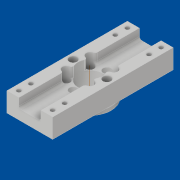
# Autodesk Inventor part: 401-flange
Saved by Autodesk Inventor 2018 (Build 220112000, 112)
## iProperties
Created: 2020-06-11
Part Number: 401-flange
Material: Generic
Document SubType Name: Modeling
Designer: Bunny320
Density: 1 g/cm^3
Appearance: Default
Author: Bunny320
Autodesk Inventor part; units mm, degrees
ref_plane "YZ Plane" through (0, 0, 0) normal (1, 0, 0) x (0, 1, 0)
ref_plane "XZ Plane" through (0, 0, 0) normal (0, 1, 0) x (-1, 0, 0)
ref_plane "XY Plane" through (0, 0, 0) normal (0, 0, 1) x (1, 0, 0)
sketch "Sketch1" plane through (0, 0, 0) normal (0, 0, 1) x (1, 0, 0)
  circle A0 centre (0, 0) radius 17.5
  dimension "d0" = 35
  constraints: 1 centre point, 1 coincident
  measures "d0" diameter of A0
extrude "Extrusion1" add sketch "Sketch1" along normal blind 5
sketch "Sketch2" plane through (0, 0, 5) normal (0, 0, 1) x (1, 0, 0)
  line L0 (-19, -50) -> (19, -50)
  line L1 (19, -50) -> (19, 50)
  line L2 (19, 50) -> (-19, 50)
  line L3 (-19, 50) -> (-19, -50)
  line L4 (-19, -50) -> (19, 50) construction
  line L5 (19, -50) -> (-19, 50) construction
  point P0 (0, 0)
  dimension "d3" = 38
  dimension "d4" = 100
  constraints: 12 end point, 2 midpoint, 2 parallel, 1 horizontal, 1 perpendicular
  measures "d3" distance of L1.end L2.end
  measures "d4" distance of L0.end L1.end
extrude "Extrusion2" add sketch "Sketch2" along normal blind 16
sketch "Sketch3" plane through (0, 0, 21) normal (0, 0, 1) x (1, 0, 0)
  point P0 (0, 0)
  point P1 (14, 0)
  dimension "d7" = 14
  constraints: 1 horizontal alignment
  measures "d7" distance of point (0, 0) point (14, 0)
hole "Hole1" at (14, 0, 21) direction (0, 0, -1) diameter 3.4 end through all counterbore diameter 6.5 counterbore depth 12 clearance for "Socket Head Cap Screw DIN EN ISO 4762" size "M3" standard "DIN"
pattern_circular "Circular Pattern1" count 8 over 360 about axis through (0, 0, -10) along (0, 0, 1) of "Hole1"
sketch "Sketch4" plane through (0, 0, 5) normal (0, 0, -1) x (-1, 0, 0)
  line L0 (-14, 45) -> (14, 45)
  line L1 (14, 45) -> (14, 35)
  line L2 (14, 35) -> (-14, 35)
  line L3 (-14, 35) -> (-14, 45)
  line L4 (-14, 45) -> (14, 35) construction
  line L5 (14, 45) -> (-14, 35) construction
  line L6 (-19, 50) -> (19, 50) projected
  line L7 (19, 50) -> (19, -50) projected
  line L8 (-19, -50) -> (-19, 50) projected
  point P0 (0, 0)
  point P1 (0, 40)
  dimension "d18" = 5
  dimension "d19" = 5
  dimension "d20" = 5
  dimension "d21" = 10
  constraints: 12 end point, 4 coincident, 2 midpoint, 2 parallel, 1 horizontal, 1 perpendicular
  measures "d18" distance between parallel lines of L6 L0
  measures "d19" distance between parallel lines of L7 L1
  measures "d20" distance between parallel lines of L8 L3
  measures "d21" distance between parallel lines of L2 L0
hole "Hole2" at (14, 45, 5) at (-14, 45, 5) at (-14, 35, 5) at (14, 35, 5) direction (0, 0, 1) diameter 3.4 end through all counterbore diameter 6.5 counterbore depth 11.4 clearance for "Socket Head Cap Screw DIN EN ISO 4762" size "M3" standard "DIN"
mirror "Mirror1" about plane through (0, 0, 0) normal (0, 1, 0) of "Hole2"
fillet "Fillet1" radius 2 1 edges at (-17.5, 0, 5)
sketch "Sketch5" plane through (-19, -50, 5) normal (0, -1, 0) x (1, 0, 0)
  line L0 (10, 16) -> (28, 16)
  line L1 (28, 16) -> (28, 8)
  line L2 (28, 8) -> (10, 8)
  line L3 (10, 8) -> (10, 16)
  line L4 (10, 16) -> (28, 8) construction
  line L5 (28, 16) -> (10, 8) construction
  line L6 (0, 16) -> (38, 16) projected
  point P0 (19, -5)
  point P1 (19, 12)
  point P2 (19, 12)
  dimension "d30" = 8
  dimension "d31" = 18
  constraints: 12 end point, 3 midpoint, 2 parallel, 1 collinear, 1 horizontal, 1 perpendicular, 1 vertical alignment
  measures "d30" distance of L0.end L1.end
  measures "d31" distance of L1.end L2.end
extrude "Extrusion3" cut sketch "Sketch5" against normal through all
sketch "Sketch6" plane through (0, 0, 21) normal (0, 0, 1) x (1, 0, 0)
  circle A0 centre (0, 0) radius 10
  line L0 (9, -6.7765) -> (9, 6.7765) projected
  dimension "d37" = 20
  constraints: 1 centre point, 1 coincident
  measures "d37" diameter of A0
extrude "Extrusion4" cut sketch "Sketch6" against normal through all
fillet "Fillet2" radius 2 8 edges at (9, 6.7765, 17) (-9, 6.7765, 17) (-9, -6.7765, 17) (9, -6.7765, 17) (9, -13.0225, 17) (-9, -13.0225, 17) (-9, 13.0225, 17) (9, 13.0225, 17)
fillet "Fillet3" radius 2 8 edges at (9.4446, -13.7756, 13) (9, -32.5164, 13) (-9.4446, -13.7756, 13) (-9, -32.5164, 13) (-9.4446, 13.7756, 13) (-9, 32.5164, 13) (9.4446, 13.7756, 13) (9, 32.5164, 13)
ref_plane "Work Plane1" through (0, 0, 0) normal (0, 1, 0) x (-1, 0, 0)
equation "\"d19\" = d18"
equation "\"d20\" = d19"
equation "\"d21\" = 2 * d18"
body "Solid1"
